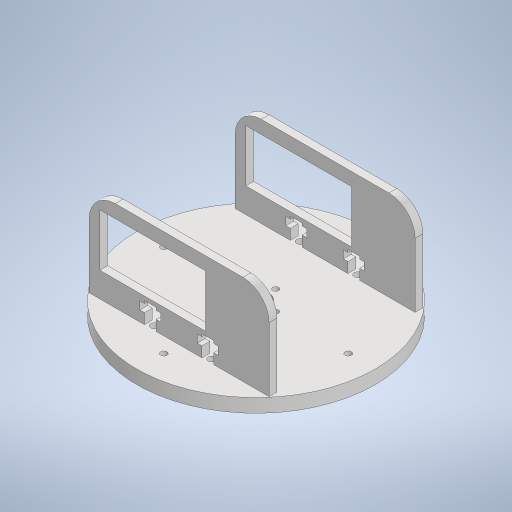
# Autodesk Inventor part: Pieza_base_2
Saved by Autodesk Inventor 2023 (Build 270158000, 158)
## iProperties
Created: 2024-09-21
Part Number: Pieza_base_2
Material: Genérico
Document SubType Name: Sheet Metal
Designer: sebas
Density: 1 g/cm^3
Sheet Metal Rule: Por defecto_mm
Appearance: Valor por defecto
Author: sebas
Autodesk Inventor part; units mm, degrees
ref_plane "YZ Plane" through (0, 0, 0) normal (1, 0, 0) x (0, 1, 0)
ref_plane "XZ Plane" through (0, 0, 0) normal (0, 1, 0) x (-1, 0, 0)
ref_plane "XY Plane" through (0, 0, 0) normal (0, 0, 1) x (1, 0, 0)
sketch "Boceto1" plane through (0, 0, 0) normal (0, 1, 0) x (-1, 0, 0)
  circle A0 centre (0, 0) radius 45.55
  dimension "d0" = 91.1
  constraints: 1 centre point, 1 coincident
  measures "d0" diameter of A0
extrude "Extrusión1" add sketch "Boceto1" along normal blind 5.2
sketch "Boceto2" plane through (0, 5.2, 0) normal (0, 1, 0) x (1, 0, 0)
  circle A0 centre (0, 0) radius 35.25 construction
  circle A1 centre (0, -35.25) radius 1.23
  dimension "d3" = 70.5
  dimension "d4" = 2.46
  constraints: 1 centre point, 1 coincident, 1 vertical alignment, 2 other
  measures "d4" diameter of A1
extrude "Extrusión2" cut sketch "Boceto2" against normal up to surface (5.2 mm away)
pattern_circular "Patrón circular1" count 4 over 360 about axis through (0, -10, 0) along (0, 1, 0) of "Extrusión2"
sketch "Boceto3" plane through (0, 0, 0) normal (0, -1, 0) x (1, 0, 0)
  line L0 (0, 0) -> (0, 27.9) construction
  line L1 (0, 27.9) -> (11, 27.9) construction
  line L2 (0, 27.9) -> (-11, 27.9) construction
  circle A0 centre (11, 27.9) radius 3.6
  circle A1 centre (-11, 27.9) radius 3.6
  dimension "d11" = 27.9
  dimension "d12" = 11
  dimension "d13" = 7.2
  dimension "d14" = 7.2
  constraints: 6 end point, 2 centre point, 2 coincident, 2 horizontal, 1 collinear, 1 vertical
  measures "d11" distance of L0.start L0.end
  measures "d12" distance of L0.end L1.end
  measures "d13" diameter of A0
  measures "d14" diameter of A1
extrude "Extrusión3" cut sketch "Boceto3" against normal blind 2.6
sketch "Boceto4" plane through (-11, 2.6, 27.9) normal (0, -1, 0) x (1, 0, 0)
  circle A0 centre (0, 0) radius 3.6 construction
  circle A1 centre (22, 0) radius 3.6 construction
  circle A2 centre (0, 0) radius 1.4
  circle A3 centre (22, 0) radius 1.4
  point P0 (11, -27.9)
  dimension "d17" = 2.8
  dimension "d18" = 2.8
  constraints: 2 centre point, 2 coincident
  measures "d17" diameter of A2
  measures "d18" diameter of A3
extrude "Extrusión4" cut sketch "Boceto4" against normal up to surface (2.6 mm away)
sketch "Boceto5" plane through (0, 5.2, 0) normal (0, 1, 0) x (1, 0, 0)
  circle A0 centre (-11, -27.9) radius 1.4 construction
  circle A1 centre (11, -27.9) radius 1.4 construction
  circle A2 centre (-11, -27.9) radius 1.4 projected
  line L0 (-11, -27.9) -> (11, -27.9) construction
  line L1 (0, 0) -> (0, -27.9) construction
  line L2 (34.4, -29.4) -> (-34.4, -29.4)
  line L3 (-34.4, -29.4) -> (-34.4, -26.4)
  line L4 (-34.4, -26.4) -> (34.4, -26.4)
  line L5 (34.4, -26.4) -> (34.4, -29.4)
  line L6 (34.4, -29.4) -> (-34.4, -26.4) construction
  line L7 (-34.4, -29.4) -> (34.4, -26.4) construction
  dimension "d21" = 68.8
  dimension "d22" = 3
  constraints: 16 end point, 3 midpoint, 2 horizontal, 2 parallel, 1 centre point, 1 perpendicular, 1 vertical
  measures "d21" distance of L3.end L4.end
  measures "d22" distance of L2.end L3.end
extrude "Extrusión5" add sketch "Boceto5" along normal blind 34.5 contours A2 | L2 L3 L4 L5
fillet "Empalme1" radius 10 2 edges at (-34.4, 39.7, 27.9) (34.4, 39.7, 27.9)
sketch "Boceto6" plane through (-34.4, 5.2, 29.4) normal (0, 0, 1) x (1, 0, 0)
  line L0 (24.8, -2.6) -> (22, -2.6) construction
  line L1 (23.4, -2.6) -> (23.4, 39) construction
  line L2 (46.8, -2.6) -> (44, -2.6) construction
  line L3 (45.4, -2.6) -> (45.4, 39) construction
  line L4 (0, 0) -> (68.8, 0) construction
  line L5 (0, 0) -> (89, 0) construction
  line L6 (25.65, 0) -> (21.15, 0)
  line L7 (21.15, 0) -> (21.15, 4)
  line L8 (21.15, 4) -> (19.4, 4)
  line L9 (19.4, 4) -> (19.4, 7)
  line L10 (27.4, 7) -> (27.4, 4)
  line L11 (27.4, 4) -> (25.65, 4)
  line L12 (25.65, 4) -> (25.65, 0)
  line L13 (21.15, 7) -> (21.15, 8)
  line L14 (21.15, 8) -> (25.65, 8)
  line L15 (25.65, 8) -> (25.65, 7)
  line L16 (19.4, 7) -> (21.15, 7)
  line L17 (25.65, 7) -> (27.4, 7)
  point P0 (34.4, -5.2)
  dimension "d26" = 8
  dimension "d27" = 4.5
  dimension "d28" = 3
  dimension "d29" = 7
  dimension "d30" = 8
  dimension "d33" = 4.5
  constraints: 30 end point, 10 perpendicular, 6 point on line, 3 vertical, 2 midpoint, 1 horizontal, 2 other
  measures "d26" distance of L9.end L10.start
  measures "d27" distance between parallel lines of L12 L7
  measures "d28" distance of L8.end L9.end
  measures "d29" distance between parallel lines of L6 L16
  measures "d30" distance between parallel lines of L6 L14
  measures "d33" distance of L13.end L14.end
extrude "Extrusión6" cut sketch "Boceto6" against normal up to surface (3 mm away)
mirror "Simetría1" about plane through (0, 0, 0) normal (1, 0, 0) of "Extrusión6"
mirror "Simetría2" about plane through (0, 0, 0) normal (0, 0, 1) of "Extrusión6", "Simetría1", "Empalme1", "Extrusión5", "Extrusión4", "Extrusión3"
sketch "Boceto7" plane through (0, 0, 0) normal (0, -1, 0) x (1, 0, 0)
  circle A0 centre (0, 0) radius 4.85
  dimension "d34" = 9.7
  constraints: 1 centre point, 1 coincident
  measures "d34" diameter of A0
extrude "Extrusión7" cut sketch "Boceto7" against normal up to surface (5.2 mm away)
sketch "Boceto8" plane through (0, 0, 0) normal (0, -1, 0) x (1, 0, 0)
  circle A0 centre (0, 0) radius 7.5 construction
  circle A1 centre (0, -7.5) radius 1.15
  dimension "d37" = 15
  dimension "d38" = 2.3
  constraints: 1 centre point, 1 coincident, 1 vertical alignment, 2 other
  measures "d38" diameter of A1
extrude "Extrusión8" cut sketch "Boceto8" against normal up to surface (5.2 mm away)
pattern_circular "Patrón circular2" count 4 over 360 about axis through (0, 0, 0) along (0, 1, 0) of "Extrusión8"
sketch "Boceto9" plane through (0, 0, 0) normal (0, -1, 0) x (1, 0, 0)
  line L0 (-31.3353, -6.1875) -> (-31.3353, 5.3887) construction
  line L1 (-31.3353, 5.3887) -> (-17.3282, 5.3887) construction
  line L2 (-17.3282, 5.3887) -> (-17.3282, -6.1875) construction
  line L3 (-17.3282, -6.1875) -> (-31.3353, -6.1875) construction
  line L4 (-16.0193, 4.1569) -> (-16.0193, -5.0935)
  line L5 (-16.0193, -5.0935) -> (-18.1465, -5.0935)
  spline S0 degree 2 poles (-18.1465, -5.0935) (-19.0825, -4.0968) (-20.8207, -2.322) (-21.7567, -1.4711) knots 0 0 0 1 2 2 2
  spline S1 degree 2 poles (-21.7567, -1.4711) (-23.6408, 0.2428) (-25.9018, 1.4948) (-27.1052, 1.4948) knots 0 0 0 1 2 2 2
  spline S2 degree 2 poles (-27.1052, 1.4948) (-27.7373, 1.4948) (-28.6854, 1.1058) (-28.9893, 0.7533) knots 0 0 0 1 2 2 2
  spline S3 degree 2 poles (-28.9893, 0.7533) (-29.2932, 0.4008) (-29.5971, -0.523) (-29.5971, -1.0822) knots 0 0 0 1 2 2 2
  spline S4 degree 2 poles (-29.5971, -1.0822) (-29.5971, -1.617) (-29.3297, -2.711) (-29.123, -3.2094) knots 0 0 0 1 2 2 2
  spline S5 degree 2 poles (-29.123, -3.2094) (-28.9528, -3.6348) (-28.4666, -4.425) (-28.2964, -4.6681) knots 0 0 0 1 2 2 2
  line L6 (-28.2964, -4.6681) -> (-28.2964, -4.7775)
  line L7 (-28.2964, -4.7775) -> (-30.4358, -4.7775)
  spline S6 degree 2 poles (-30.4358, -4.7775) (-30.7397, -4.1575) (-31.3353, -1.9331) (-31.3353, -0.9363) knots 0 0 0 1 2 2 2
  spline S7 degree 2 poles (-31.3353, -0.9363) (-31.3353, 1.1666) (-29.1109, 3.537) (-27.2146, 3.537) knots 0 0 0 1 2 2 2
  spline S8 degree 2 poles (-27.2146, 3.537) (-26.3272, 3.537) (-24.8442, 3.1237) (-24.2121, 2.759) knots 0 0 0 1 2 2 2
  spline S9 degree 2 poles (-24.2121, 2.759) (-23.5557, 2.3943) (-22.2673, 1.3368) (-21.6473, 0.7533) knots 0 0 0 1 2 2 2
  spline S10 degree 2 poles (-21.6473, 0.7533) (-20.6141, -0.1948) (-18.4018, -2.5165) (-17.7575, -3.2094) knots 0 0 0 1 2 2 2
  line L8 (-17.7575, -3.2094) -> (-17.7575, 4.1569)
  line L9 (-17.7575, 4.1569) -> (-16.0193, 4.1569)
  point P0 (0, 0)
  constraints: 2 other
extrude "Extrusión9" cut sketch "Boceto9" against normal blind 0.5
sketch "Boceto10" plane through (-24.4, 39.7, 29.4) normal (0, 0, 1) x (1, 0, 0)
  circle A0 centre (5, -15) radius 2.5
  line L0 (-10, -34.5) -> (-10, -10) construction
  line L1 (0, 0) -> (48.8, 0) construction
  point P0 (24.4, -39.7)
  dimension "d46" = 5
  dimension "d47" = 15
  dimension "d48" = 15
  constraints: 1 centre point
  measures "d46" diameter of A0
  measures "d47" distance from line of L0 A0.centre
  measures "d48" distance from line of L1 A0.centre
extrude "Extrusión10" cut sketch "Boceto10" against normal up to surface (58.8 mm away)
sketch "Boceto11" plane through (-24.4, 39.7, 29.4) normal (0, 0, 1) x (1, 0, 0)
  line L0 (-5.9, -5) -> (34.5, -5)
  line L1 (34.5, -5) -> (34.5, -25)
  line L2 (34.5, -25) -> (-5.9, -25)
  line L3 (-5.9, -25) -> (-5.9, -5)
  line L4 (0, 0) -> (48.8, 0) projected
  point P0 (24.4, -39.7)
  dimension "d51" = 40.4
  dimension "d52" = 20
  dimension "d53" = 5
  constraints: 8 end point, 2 parallel, 1 horizontal, 1 perpendicular
  measures "d51" distance of L1.end L2.end
  measures "d52" distance of L0.end L1.end
  measures "d53" distance between parallel lines of L4 L0
extrude "Extrusión11" cut sketch "Boceto11" against normal up to surface (58.8 mm away)
equation "\"Radio_pliegue\" = Grosor"
equation "\"Anchura_desahogo_plegado\" = Grosor"
equation "\"Profundidad_desahogo_plegado\" = 0.5 * Grosor"
equation "\"Tamaño_destalonado\" = 4 * Grosor"
equation "\"Remanente_mínimo\" = 2 * Grosor"
equation "\"Radiodetransición\" = Radio_pliegue"
equation "\"Tamaño_de_radio_de_Jacobi\" = Radio_pliegue"
equation "\"TamañoSeparación\" = Grosor"
equation "\"Grosor\" = 0.5"
